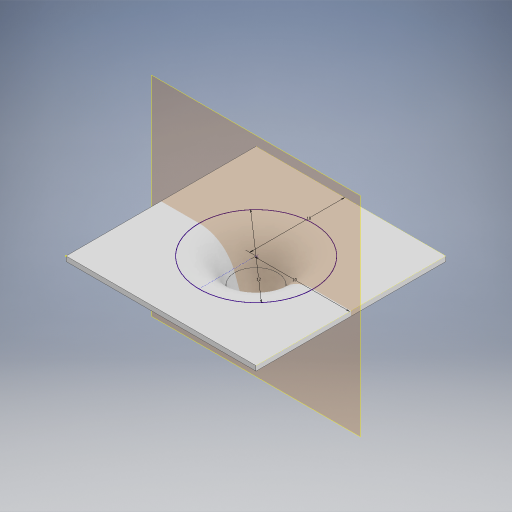
# Autodesk Inventor part: CE-4.1.1
Saved by Autodesk Inventor 2024 (Build 280153000, 153)
## iProperties
Created: 2024-02-07
Part Number: CE-4.1.1
Material: Generic
Document SubType Name: Sheet Metal
Designer: Alex
Density: 1 g/cm^3
Sheet Metal Rule: Default_mm
Appearance: Default
Author: Alex
Autodesk Inventor part; units mm, degrees
ref_plane "YZ Plane" through (0, 0, 0) normal (1, 0, 0) x (0, 1, 0)
ref_plane "XZ Plane" through (0, 0, 0) normal (0, 1, 0) x (-1, 0, 0)
ref_plane "XY Plane" through (0, 0, 0) normal (0, 0, 1) x (1, 0, 0)
sketch "Sketch5" plane through (0, 0, 0) normal (0, 1, 0) x (-1, 0, 0)
  line L0 (0, 0) -> (-20, 0)
  line L1 (-20, 0) -> (-20, -20)
  line L2 (-20, -20) -> (0, -20)
  line L3 (0, -20) -> (0, 0)
  dimension "d13" = 20
  measures "d13" distance of L2.end L1.end
extrude "Plate2" add sketch "Sketch5" along normal blind 0.5
sketch "Sketch6" plane through (0, 0.5, 0) normal (0, 1, 0) x (1, 0, 0)
  circle A0 centre (10, 10) radius 6
  line L0 (0, 20) -> (20, 20) construction
  line L1 (20, 20) -> (20, 0) construction
  line L2 (10, 10) -> (10, 4) construction
  point P0 (0, 0)
  dimension "d15" = 12
  dimension "d16" = 10
  dimension "d17" = 10
  constraints: 2 end point, 1 vertical, 1 vertical alignment, 2 other
  measures "d16" distance from line of L0 L2.start
  measures "d17" distance from line of L2.start L1
extrude "Extrusion2" cut sketch "Sketch6" against normal blind 0.5
ref_plane "Work Plane2" through (10, 0.5, -10) normal (0, 0, 1) x (1, 0, 0)
sketch "Sketch7" plane through (10, 0.5, -10) normal (0, 0, 1) x (1, 0, 0)
  line L0 (6, 0) -> (-6, 0) projected
  arc A0 (-2.2412, -2.6319) -> (-6, 0) centre (-6, -4) ccw
  line L1 (0, 0) -> (0, -5) construction
  line L2 (-2.2412, -2.6319) -> (-1.3793, -5)
  line L3 (-1.3793, -5) -> (-1.8492, -5.171)
  line L4 (-1.8492, -5.171) -> (-2.7111, -2.8029)
  line L5 (-6, 0) -> (-6, -0.5)
  arc A1 (-2.7111, -2.8029) -> (-6, -0.5) centre (-6, -4) ccw
  point P0 (-10, -0.5)
  dimension "d20" = 5
  dimension "d21" = 20
  dimension "d22" = 4
  dimension "d23" = 0.5
  constraints: 10 end point, 4 point on circle, 3 tangent, 2 centre point, 2 perpendicular, 2 vertical, 1 concentric, 1 horizontal alignment
  measures "d20" distance of L1.start L1.end
  measures "d21" angle of L2 L1
  measures "d22" radius of A0
  measures "d23" distance between parallel lines of L4 L2
revolve "Revolution2" add sketch "Sketch7" angle 360 about axis through (10, 0.5, -10) along (0, -1, 0)
equation "\"d18\" = Thickness"
equation "\"d23\" = Thickness"
equation "\"d14\" = Thickness"
equation "\"BendRadius\" = Thickness"
equation "\"BendReliefWidth\" = Thickness"
equation "\"BendReliefDepth\" = 0.5 * Thickness"
equation "\"CornerReliefSize\" = 4 * Thickness"
equation "\"MinimumRemnant\" = 2 * Thickness"
equation "\"TransitionRadius\" = BendRadius"
equation "\"JacobiRadiusSize\" = BendRadius"
equation "\"GapSize\" = Thickness"
equation "\"Thickness\" = 0.5"
body "Solid2"
